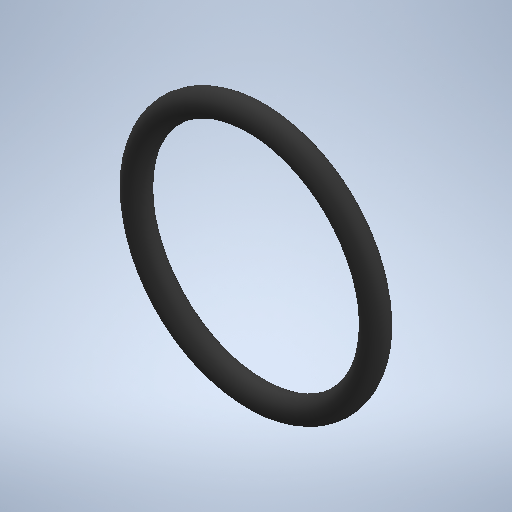
# Autodesk Inventor part: O-ring_D63
Saved by Autodesk Inventor 2025.3 (Build 293356030, 356C)
## iProperties
Created: 2025-09-06
Part Number: O-ring_D63
Material: 一般
Document SubType Name: Modeling
Designer: daisuke
Density: 1 g/cm^3
Appearance: ゴム - 黒
Author: daisuke
Autodesk Inventor part; units mm, degrees
ref_plane "YZ Plane" through (0, 0, 0) normal (1, 0, 0) x (0, 1, 0)
ref_plane "XZ Plane" through (0, 0, 0) normal (0, 1, 0) x (-1, 0, 0)
ref_plane "XY Plane" through (0, 0, 0) normal (0, 0, 1) x (1, 0, 0)
sketch "スケッチ1" plane through (0, 0, 0) normal (0, 1, 0) x (-1, 0, 0)
  line L0 (0, 0) -> (-103.3594, 0) construction
  circle A0 centre (0, 0) radius 25.8 construction
  circle A1 centre (0, 0) radius 31.5 construction
  line L1 (-31.5, -14.3346) -> (-31.5, 14.3346) construction
  line L2 (-28.65, 17.2911) -> (-28.65, -17.2911) construction
  line L3 (-25.8, -14.4815) -> (-25.8, 14.4815) construction
  circle A2 centre (-28.65, 0) radius 2.85
  line L4 (0, -44.1) -> (0, 44.1) projected
  point P0 (-31.5, 0)
  point P1 (-25.8, 0)
  dimension "d0" = 51.6
  dimension "d1" = 63
  constraints: 8 end point, 3 centre point, 3 coincident, 3 midpoint, 3 point on line, 3 tangent, 2 vertical, 1 horizontal, 1 other
  measures "d0" diameter of A0
  measures "d1" diameter of A1
revolve "回転1" add sketch "スケッチ1" angle 360 about axis through (0, 0, -10) along (0, 0, 1)
